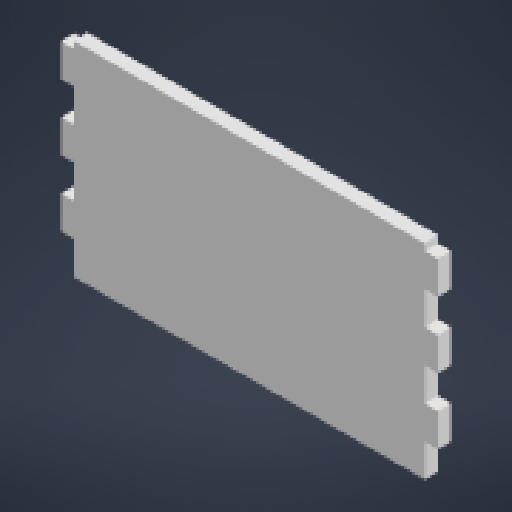
# Autodesk Inventor part: стульчак 4
Saved by Autodesk Inventor 2025 (Build 290162000, 162)
## iProperties
Created: 2025-01-29
Part Number: стульчак 4
Material: Типовые
Document SubType Name: Modeling
Designer: Phantom
Density: 1 g/cm^3
Appearance: По умолчанию
Author: Phantom
Autodesk Inventor part; units mm, degrees
ref_plane "YZ Plane" through (0, 0, 0) normal (1, 0, 0) x (0, 1, 0)
ref_plane "XZ Plane" through (0, 0, 0) normal (0, 1, 0) x (-1, 0, 0)
ref_plane "XY Plane" through (0, 0, 0) normal (0, 0, 1) x (1, 0, 0)
sketch "Эскиз1" plane through (0, 0, 0) normal (0, 0, 1) x (1, 0, 0)
  line L0 (0, 0) -> (106.3, 0)
  line L1 (106.3, 0) -> (106.3, 62)
  line L2 (106.3, 62) -> (0, 62)
  line L3 (0, 62) -> (0, 0)
  dimension "d0" = 106.3
  dimension "d1" = 62
  constraints: 8 end point, 2 parallel, 1 horizontal, 1 perpendicular
  measures "d0" distance of L2.end L1.end
  measures "d1" distance of L1.end L0.end
extrude "Выдавливание1" add sketch "Эскиз1" along normal blind 4
sketch "Эскиз2" plane through (0, 0, 4) normal (0, 0, 1) x (1, 0, 0)
  line L0 (106.3, 10) -> (106.3, 20) projected
  line L1 (110.3, 10) -> (106.3, 10) projected
  line L2 (110.3, 20) -> (110.3, 10) projected
  line L3 (110.3, 20) -> (106.3, 20) projected
  line L4 (106.3, 30) -> (106.3, 40) projected
  line L5 (110.3, 30) -> (106.3, 30) projected
  line L6 (110.3, 40) -> (110.3, 30) projected
  line L7 (110.3, 40) -> (106.3, 40) projected
  line L8 (106.3, 50) -> (106.3, 60) projected
  line L9 (110.3, 50) -> (106.3, 50) projected
  line L10 (110.3, 60) -> (110.3, 50) projected
  line L11 (110.3, 60) -> (106.3, 60) projected
  line L12 (-4, 10) -> (-4, 20) projected
  line L13 (0, 10) -> (-4, 10) projected
  line L14 (0, 20) -> (0, 10) projected
  line L15 (0, 20) -> (-4, 20) projected
  line L16 (-4, 30) -> (-4, 40) projected
  line L17 (0, 30) -> (-4, 30) projected
  line L18 (0, 40) -> (0, 30) projected
  line L19 (0, 40) -> (-4, 40) projected
  line L20 (-4, 50) -> (-4, 60) projected
  line L21 (0, 50) -> (-4, 50) projected
  line L22 (0, 60) -> (0, 50) projected
  line L23 (0, 60) -> (-4, 60) projected
  point P0 (0, 0)
extrude "Выдавливание2" add sketch "Эскиз2" against normal up to surface (4 mm away)
sketch "Эскиз3" plane through (-4, 50, 4) normal (-1, 0, 0) x (0, 0, 1)
  line L0 (-4, 10) -> (0, 10) projected
  line L1 (0, 10) -> (0, 16) projected
  line L2 (0, 16) -> (-10, 16.6879) projected
  line L3 (-10, 16.6879) -> (-10, 12.6879) projected
  line L4 (-10, 12.6879) -> (-20, 13.3759) projected
  line L5 (-20, 13.3759) -> (-20, 17.3759) projected
  line L6 (-20, 17.3759) -> (-30, 18.0638) projected
  line L7 (-30, 18.0638) -> (-30, 14.0638) projected
  line L8 (-30, 14.0638) -> (-40, 14.7517) projected
  line L9 (-40, 14.7517) -> (-40, 18.7517) projected
  line L10 (-40, 18.7517) -> (-50, 19.4397) projected
  line L11 (-50, 19.4397) -> (-50, 15.4397) projected
  line L12 (-50, 15.4397) -> (-60, 16.1276) projected
  line L13 (-60, 16.1276) -> (-60, 20.1276) projected
  line L14 (-60, 20.1276) -> (-70, 20.8155) projected
  line L15 (-70, 20.8155) -> (-70, 16.8155) projected
  line L16 (-70, 16.8155) -> (-80, 17.5035) projected
  line L17 (-80, 17.5035) -> (-80, 21.5035) projected
  line L18 (-80, 21.5035) -> (-90, 22.1914) projected
  line L19 (-90, 22.1914) -> (-90, 18.1914) projected
  line L20 (-90, 18.1914) -> (-100, 18.8794) projected
  line L21 (-100, 18.8794) -> (-100, 22.8794) projected
  line L22 (-100, 22.8794) -> (-110, 23.5673) projected
  line L23 (-110, 23.5673) -> (-110, 19.5673) projected
  line L24 (-110, 19.5673) -> (-120, 20.2552) projected
  line L25 (-120, 20.2552) -> (-120, 24.2552) projected
  line L26 (-120, 24.2552) -> (-130, 24.9432) projected
  line L27 (-130, 24.9432) -> (-130, 20.9432) projected
  line L28 (-130, 20.9432) -> (-140, 21.6311) projected
  line L29 (-140, 21.6311) -> (-140, 25.6311) projected
  line L30 (-140, 25.6311) -> (-145.3625, 26) projected
  line L31 (-145.3625, 26) -> (-145.3625, 16) projected
  line L32 (-145.3625, 16) -> (-208, -30) projected
  line L33 (-208, -50) -> (-208, -30) projected
  line L34 (-187, -50) -> (-208, -50) projected
  line L35 (-187, -54) -> (-187, -50) projected
  line L36 (-177, -54) -> (-187, -54) projected
  line L37 (-177, -50) -> (-177, -54) projected
  line L38 (-167, -50) -> (-177, -50) projected
  line L39 (-167, -54) -> (-167, -50) projected
  line L40 (-157, -54) -> (-167, -54) projected
  line L41 (-157, -50) -> (-157, -54) projected
  line L42 (-147, -50) -> (-157, -50) projected
  line L43 (-147, -54) -> (-147, -50) projected
  line L44 (-137, -54) -> (-147, -54) projected
  line L45 (-137, -50) -> (-137, -54) projected
  line L46 (-127, -50) -> (-137, -50) projected
  line L47 (-127, -54) -> (-127, -50) projected
  line L48 (-117, -54) -> (-127, -54) projected
  line L49 (-117, -50) -> (-117, -54) projected
  line L50 (-107, -50) -> (-117, -50) projected
  line L51 (-107, -54) -> (-107, -50) projected
  line L52 (-97, -54) -> (-107, -54) projected
  line L53 (-97, -50) -> (-97, -54) projected
  line L54 (-87, -50) -> (-97, -50) projected
  line L55 (-87, -54) -> (-87, -50) projected
  line L56 (-77, -54) -> (-87, -54) projected
  line L57 (-77, -50) -> (-77, -54) projected
  line L58 (-67, -50) -> (-77, -50) projected
  line L59 (-67, -54) -> (-67, -50) projected
  line L60 (-57, -54) -> (-67, -54) projected
  line L61 (-57, -50) -> (-57, -54) projected
  line L62 (-47, -50) -> (-57, -50) projected
  line L63 (-47, -54) -> (-47, -50) projected
  line L64 (-37, -54) -> (-47, -54) projected
  line L65 (-37, -50) -> (-37, -54) projected
  line L66 (-27, -50) -> (-37, -50) projected
  line L67 (-27, -54) -> (-27, -50) projected
  line L68 (-17, -54) -> (-27, -54) projected
  line L69 (-17, -50) -> (-17, -54) projected
  line L70 (-17, -50) -> (0, -50) projected
  line L71 (0, -50) -> (0, -40) projected
  line L72 (0, -40) -> (-4, -40) projected
  line L73 (-4, -40) -> (-4, -30) projected
  line L74 (-4, -30) -> (0, -30) projected
  line L75 (0, -30) -> (0, -20) projected
  line L76 (0, -20) -> (-4, -20) projected
  line L77 (-4, -20) -> (-4, -10) projected
  line L78 (-4, -10) -> (0, -10) projected
  line L79 (0, -10) -> (0, 0) projected
  line L80 (0, 0) -> (-4, 0) projected
  line L81 (-4, 0) -> (-4, 10) projected
  line L82 (-4, 12) -> (0, 12) projected
  line L83 (0, 12) -> (-10, 12.6879) projected
  line L84 (-4, 12) -> (-4, 13.5119)
  point P0 (-4, -50)
  point P1 (-4, 12.2752)
  constraints: 2 end point, 1 vertical
extrude "Выдавливание3" add sketch "Эскиз3" against normal up to surface (110.3 mm away) contours L82 L84 L83
sketch "Эскиз4" plane through (-4, 50, 4) normal (-1, 0, 0) x (0, 0, 1)
  line L0 (-4, 12) -> (0, 12) projected
  line L1 (0, 12) -> (-4, 12.2752) projected
  line L2 (-4, 12.2752) -> (-4, 12) projected
  point P0 (-4, -50)
extrude "Выдавливание4" cut sketch "Эскиз4" against normal up to surface (4 mm away)
